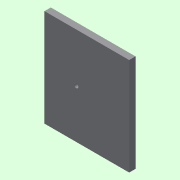
# Autodesk Inventor part: Distance_test_adaptor_circle_1mm
Saved by Autodesk Inventor 2015 (Build 190159000, 159)
## iProperties
Created: 2015-05-18
Part Number: Distance_test_adaptor_circle_1mm
Material: Generic
Document SubType Name: Modeling
Designer: Openlab
Density: 1 g/cm^3
Appearance: Default
Author: Openlab
Autodesk Inventor part; units mm, degrees
ref_plane "YZ Plane" through (0, 0, 0) normal (1, 0, 0) x (0, 1, 0)
ref_plane "XZ Plane" through (0, 0, 0) normal (0, 1, 0) x (-1, 0, 0)
ref_plane "XY Plane" through (0, 0, 0) normal (0, 0, 1) x (1, 0, 0)
sketch "Sketch1" plane through (0, 0, 0) normal (0, 1, 0) x (-1, 0, 0)
  line L0 (0, 0) -> (0, -23)
  line L1 (0, -23) -> (20, -23)
  line L2 (20, -23) -> (20, 0)
  line L3 (16.0214, -11.5) -> (3.8301, -11.5) construction
  circle A0 centre (12.5, -11.5) radius 0.5
  line L4 (20, 0) -> (0, 0)
  dimension "d0" = 23
  dimension "d2" = 1
  dimension "d3" = 7.5
  dimension "d10" = 20
  constraints: 10 end point, 2 horizontal, 1 centre point, 1 perpendicular, 1 point on line, 1 vertical, 1 other
  measures "d0" distance of L0.end L0.start
  measures "d2" diameter of A0
  measures "d3" distance from line of L2 A0.centre
  measures "d10" distance of L2.end L0.start
extrude "Extrusion3" add sketch "Sketch1" along normal blind 1.5
body "Solid2"
